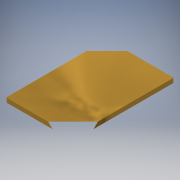
# Autodesk Inventor part: lámina
Saved by Autodesk Inventor 2016 (Build 200138000, 138)
## iProperties
Created: 2015-11-12
Part Number: lámina
Material: Latón, amarillo claro
Document SubType Name: Chapa
Designer: David
Density: 8.47 g/cm^3
Sheet Metal Rule: Por defecto_mm
Appearance: Latón - Satinado
Author: David
Autodesk Inventor part; units mm, degrees
note: some values were not read from the file. Chosen so that the rebuilt part matches the saved one: relief shape of "Placa2".
ref_plane "YZ Plane" through (0, 0, 0) normal (1, 0, 0) x (0, 1, 0)
ref_plane "XZ Plane" through (0, 0, 0) normal (0, 1, 0) x (-1, 0, 0)
ref_plane "XY Plane" through (0, 0, 0) normal (0, 0, 1) x (1, 0, 0)
sketch "Boceto1" plane through (0, 0, 0) normal (0, 0, 1) x (1, 0, 0)
  line L0 (-19.05, -19.05) -> (-19.05, 19.05)
  line L1 (19.05, -19.05) -> (-19.05, -19.05)
  line L2 (-14.2875, 16.764) -> (-14.2875, -9.4615)
  line L3 (-9.4615, -14.2875) -> (16.764, -14.2875)
  arc A0 (-14.2875, -9.4615) -> (-9.4615, -14.2875) centre (-9.4615, -9.4615) ccw
  line L4 (-14.2875, -9.4615) -> (-14.2875, 871.3615)
  line L5 (-9.4615, 876.1875) -> (571.3615, 876.1875)
  line L6 (576.1875, 871.3615) -> (576.1875, -9.4615)
  line L7 (571.3615, -14.2875) -> (-9.4615, -14.2875)
  arc A1 (571.3615, -14.2875) -> (576.1875, -9.4615) centre (571.3615, -9.4615) ccw
  arc A2 (576.1875, 871.3615) -> (571.3615, 876.1875) centre (571.3615, 871.3615) ccw
  arc A3 (-9.4615, 876.1875) -> (-14.2875, 871.3615) centre (-9.4615, 871.3615) ccw
  line L8 (-14.2875, -9.4615) -> (-14.2875, -9.4615)
  arc A4 (-14.2875, -9.4615) -> (-9.4615, -14.2875) centre (-9.4615, -9.4615) ccw
  point P0 (0, 0)
  point P1 (-14.2875, -14.2875)
  point P2 (-14.2875, 876.1875)
  point P3 (576.1875, 876.1875)
  point P4 (576.1875, -14.2875)
  dimension "d3" = 890.475
  dimension "d5" = 890.475
  dimension "d6" = 4.826
  dimension "d7" = 4.826
  dimension "d8" = 4.826
  dimension "d9" = 4.826
  measures "d3" distance of point (-14.287, -14.288) point (-14.288, 876.187)
  measures "d5" distance of point (576.187, 876.187) point (576.187, -14.288)
  measures "d6" radius of A0
  measures "d7" radius of A1
  measures "d8" radius of A2
  measures "d9" radius of A4
sketch "Boceto1 outline for Placa1" plane through (0, 0, 0) normal (0, 0, 1) x (1, 0, 0)
  line L0 (-14.2875, -9.4615) -> (-14.2875, 871.3615)
  arc A0 (-14.2875, 871.3615) -> (-9.4615, 876.1875) centre (-9.4615, 871.3615) cw
  line L1 (-9.4615, 876.1875) -> (571.3615, 876.1875)
  arc A1 (571.3615, 876.1875) -> (576.1875, 871.3615) centre (571.3615, 871.3615) cw
  line L2 (576.1875, 871.3615) -> (576.1875, -9.4615)
  arc A2 (576.1875, -9.4615) -> (571.3615, -14.2875) centre (571.3615, -9.4615) cw
  line L3 (571.3615, -14.2875) -> (-9.4615, -14.2875)
  arc A3 (-9.4615, -14.2875) -> (-14.2875, -9.4615) centre (-9.4615, -9.4615) cw
extrude "Placa1" add sketch "Boceto1 outline for Placa1" along normal blind 1
sketch "Boceto2" plane through (-9.4615, -13.2875, 1) normal (0, -1, 0) x (1, 0, 0)
  line L0 (580.823, 0) -> (0, 0)
  line L1 (0, 0) -> (0, -38.1)
  line L2 (0, -38.1) -> (580.823, -38.1)
  line L3 (580.823, -38.1) -> (580.823, 0)
  constraints: 6 end point, 1 horizontal, 1 perpendicular, 1 vertical
edge flange "Pestaña1" height 38.1 angle 90 thickness 1 bend radius 1 thickness toward (0, -1, 0) relief straight relief width 1 relief depth 0.5 corner gap 1 corner form 0 edges at (280.95, -14.2875, 0) (-14.2875, 430.95, 0) (280.95, 876.1875, 0) (576.1875, 430.95, 0) wall of the first edge with corners at (571.3615, -13.2875, 1) (-9.4615, -13.2875, 1) (-9.4615, -13.2875, -37.1) (571.3615, -13.2875, -37.1)
bend "Doblez1"
corner "Esquina1"
equation "\"d10\" = Anchura_desahogo_plegado"
equation "\"d11\" = Profundidad_desahogo_plegado"
equation "\"d12\" = Remanente_mínimo"
equation "\"d13\" = Radio_pliegue"
equation "\"d16\" = Radio_pliegue"
equation "\"d17\" = Tamaño_destalonado"
equation "\"d18\" = TamañoSeparación"
equation "\"d19\" = Tamaño_de_radio_de_Jacobi"
equation "\"Radio_pliegue\" = Grosor"
equation "\"Anchura_desahogo_plegado\" = Grosor"
equation "\"Profundidad_desahogo_plegado\" = 0.5 * Grosor"
equation "\"Tamaño_destalonado\" = 4 * Grosor"
equation "\"Remanente_mínimo\" = 2 * Grosor"
equation "\"Radiodetransición\" = Radio_pliegue"
equation "\"Tamaño_de_radio_de_Jacobi\" = Radio_pliegue"
equation "\"TamañoSeparación\" = Grosor"
equation "\"d2\" = Radio_pliegue"
equation "\"Grosor\" = 1"
